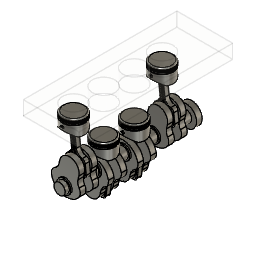
ic engine (Autodesk Fusion 360 design; units mm, degrees)
part number: 2025-07-07-10-14-35-876
part number: 2025-07-07-10-17-05-050
part number: 2025-07-07-10-17-21-308
part number: 2025-07-07-10-30-57-029
part number: 2025-07-07-10-31-19-349
part number: 2025-07-07-10-58-43-578
part number: 2025-07-07-10-58-53-469
part number: 2025-07-07-11-04-14-439
part number: 2025-07-07-15-54-50-928
part number: 2025-07-07-16-06-10-708
part number: 2025-07-07-16-45-22-649
Autodesk Fusion 360 part; units mm, degrees
note: some values were not read from the file. Set by a fixed rule: which face or edge a step refers to.
sketch "Sketch1" plane through (0, 0, 0) normal (0, 1, 0) x (1, 0, 0) in component "PISTON"
  line L0 (0, 0) -> (40, 0)
  line L1 (40, 0) -> (40, -55)
  line L2 (40, -55) -> (0, -55)
  line L3 (0, -55) -> (0, 0)
  line L4 (40, -48) -> (36, -48)
  line L5 (36, -48) -> (36, -46)
  line L6 (36, -46) -> (40, -46)
  line L7 (40, -46) -> (40, -48)
  line L8 (40, -44) -> (36, -44)
  line L9 (36, -44) -> (36, -42)
  line L10 (36, -42) -> (40, -42)
  line L11 (40, -42) -> (40, -44)
  line L12 (40, -38) -> (36, -38)
  line L13 (36, -38) -> (36, -36)
  line L14 (36, -36) -> (40, -36)
  line L15 (40, -36) -> (40, -38)
  dimension "d1" = 40
  dimension "d2" = 55
  dimension "d3" = 2
  dimension "d4" = 2
  dimension "d5" = 2
  dimension "d6" = 7
  dimension "d7" = 4
  dimension "d8" = 4
  dimension "d9" = 4
  dimension "d10" = 2
  dimension "d11" = 4
  constraint horizontal L0
  constraint vertical L1
  constraint horizontal L2
  constraint vertical L3
  constraint coincident L0.start L3.end
  constraint horizontal L4
  constraint vertical L5
  constraint horizontal L6
  constraint vertical L7
  constraint coincident L1 L4.start
  constraint horizontal L8
  constraint vertical L9
  constraint horizontal L10
  constraint vertical L11
  constraint coincident L1 L8.start
  constraint horizontal L12
  constraint vertical L13
  constraint horizontal L14
  constraint vertical L15
  constraint coincident L1 L12.start
  measures "d1" distance of L0.start L0.end
  measures "d2" distance of L0.start L2.end
  measures "d3" distance of L4.end L5.end
  measures "d4" distance of L8.end L9.end
  measures "d5" distance of L12.end L13.end
  measures "d6" distance of L2 L4
  measures "d7" distance of L4.start L4.end
  measures "d8" distance of L8.start L8.end
  measures "d9" distance of L12.start L12.end
  measures "d10" distance of L6 L8
  measures "d11" distance of L10 L12
revolve "Revolve1" add sketch "Sketch1" angle 360 about axis through (0, 0, 55) along (0, 0, -1) contours L0 L1 L2 L3 L4 L5 L6 L8 L9 L10 L12 L13 L14 makes body 1 in component "PISTON"
fillet "Fillet1" radius 5 1 edges at (-37.2931, -14.4646, 55) on bodies 1 in component "PISTON"
sketch "Sketch2" plane through (0, 0, 0) normal (0, 0, -1) x (1, 0, 0) in component "PISTON"
  circle A0 centre (0, 0) radius 40
  circle A1 centre (0, 0) radius 35
  dimension "d15" = 70
  constraint coincident A0.centre A1.centre
  measures "d15" diameter of A1
extrude "Extrude1" cut sketch "Sketch2" against normal blind 50 contours A1 bodies 1 in component "PISTON"
sketch "Sketch3" plane through (0, 0, 0) normal (0, 1, 0) x (1, 0, 0) in component "PISTON"
  line L0 (-40, 0) -> (40, 0)
  line L1 (-40, -36) -> (40, -36)
  line L2 (0, 0) -> (0, -13.6111)
  arc A0 (-35.5, 0) -> (35.5, 0) centre (0, 39.4894) ccw
  circle A1 centre (0, -24) radius 5
  dimension "d18" = 10
  dimension "d19" = 4.5
  dimension "d20" = 4.5
  dimension "d21" = 24
  constraint coincident L2.start origin
  constraint perpendicular L0 L2
  constraint coincident L2.end A0
  constraint coincident L0 A0.start
  constraint coincident L0 A0.end
  measures "d18" diameter of A1
  measures "d19" distance of L0.end A0.end
  measures "d20" distance of L0.start A0.start
  measures "d21" distance of L2.start A1.centre
extrude "Extrude2" cut sketch "Sketch3" along normal mid plane 80 bodies 1 in component "PISTON"
pattern_linear "00000000-0000-0000-0000-000000000000" [suppressed] in component "PISTONS"
sketch "Sketch1 (2)" plane through (0, 0, 0) normal (0, 1, 0) x (1, 0, 0) in component "connecting rod"
  circle A0 centre (0, -20) radius 5
  circle A1 centre (0, -20) radius 8.5
  circle A2 centre (0, 105) radius 22.5
  line L0 (-8.5, -20) -> (-8.5, 55)
  line L1 (0, 105) -> (-36, 105)
  line L2 (-36, 105) -> (-36, 80)
  line L3 (-36, 80) -> (-33.5, 80)
  line L4 (8.5, -20) -> (8.5, 55)
  line L5 (33.5, 80) -> (36, 80)
  line L6 (36, 80) -> (36, 105)
  line L7 (36, 105) -> (0, 105)
  arc A3 (-8.5, 55) -> (-33.5, 80) centre (-33.5, 55) ccw
  arc A4 (33.5, 80) -> (8.5, 55) centre (33.5, 55) ccw
  line L8 (36, 105) -> (-36, 105)
  line L9 (-36, 105) -> (-36, 137.5)
  line L10 (-36, 137.5) -> (36, 137.5)
  line L11 (36, 137.5) -> (36, 105)
  circle A5 centre (0, -5) radius 4.75
  circle A6 centre (0, 67.5) radius 4.75
  line L12 (4.75, -5) -> (4.75, 67.5)
  line L13 (-4.75, -5) -> (-4.75, 67.5)
  point P0 (8.5, 80)
  dimension "d28" = 10
  dimension "d29" = 17
  dimension "d30" = 45
  dimension "d31" = 125
  dimension "d32" = 36
  dimension "d33" = 25
  dimension "d34" = 27.5
  dimension "d35" = 25
  dimension "d36" = 72
  dimension "d37" = 32.5
  dimension "d38" = 9.5
  dimension "d39" = 9.5
  dimension "d40" = 15
  dimension "d41" = 37.5
  constraint concentric A0 A1
  constraint coincident A1 L0.start
  constraint tangent A1 L0
  constraint vertical L0
  constraint coincident A2.centre L1.start
  constraint horizontal L1
  constraint perpendicular L1 L2
  constraint perpendicular L2 L3
  constraint coincident A1 L4.start
  constraint tangent A1 L4
  constraint vertical L4
  constraint perpendicular L4 L5
  constraint perpendicular L5 L6
  constraint perpendicular L6 L7
  constraint tangent L3 A3
  constraint tangent L0 A3
  constraint coincident P0 L4
  constraint coincident P0 L5
  constraint tangent L4 A4
  constraint tangent L5 A4
  constraint equal A3 A4
  constraint horizontal L8
  constraint vertical L9
  constraint horizontal L10
  constraint vertical L11
  constraint coincident A5 L12.start
  constraint coincident A6 L12.end
  constraint tangent A6 L12
  constraint parallel L4 L12
  constraint coincident A5 L13.start
  constraint coincident A6 L13.end
  constraint tangent A6 L13
  constraint parallel L12 L13
  measures "d28" diameter of A0
  measures "d29" diameter of A1
  measures "d30" diameter of A2
  measures "d31" distance of A0.centre A2.centre
  measures "d32" distance of A2.centre L1.end
  measures "d33" distance of L1.end L2.end
  measures "d34" distance of P0 L5.end
  measures "d35" radius of A3
  measures "d36" distance of L6.end L1.end
  measures "d37" distance of L6.end L10.end
  measures "d38" diameter of A5
  measures "d39" diameter of A6
  measures "d40" distance of A0.centre A5.centre
  measures "d41" distance of A2.centre A6.centre
extrude "Extrude1'" add sketch "Sketch1 (2)" along normal mid plane 20 separate body contours A1 | A1 A2 L0 L1 L2 L3 L4 L5 L6 L7 A3 A4 L8 | A2 L1 L7 L8 L9 L10 L11 makes body 2 in component "connecting rod"
extrude "Extrude2'" add sketch "Sketch1 (2)" along normal mid plane 10 contours A5 | A5 A6 L12 L13 | A6 bodies 2 in component "connecting rod"
fillet "Fillet1'" radius 12.5 4 edges at (36, 0, -80) (36, 0, -137.5) (-36, 0, -137.5) (-36, 0, -80) on bodies 2 in component "connecting rod"
fillet "Fillet2" radius 2.5 24 edges at (0, 10, 28.5) (8.5, 10, -17.5) (13.6044, 10, -70.1383) (33.4478, 10, -83.573) (36, 10, -108.071) (32.3388, 10, -133.8388) (0, 10, -137.5) (-32.3388, 10, -133.8388) (-36, 10, -108.071) (-33.4478, 10, -83.573) (-13.6044, 10, -70.1383) (-8.5, 10, -17.5) (-33.4478, -10, -83.573) (-36, -10, -108.071) (-32.3388, -10, -133.8388) (0, -10, -137.5) (32.3388, -10, -133.8388) (36, -10, -108.071) (33.4478, -10, -83.573) (13.6044, -10, -70.1383) (8.5, -10, -17.5) (0, -10, 28.5) (-8.5, -10, -17.5) (-13.6044, -10, -70.1383) on bodies 2 in component "connecting rod"
cylinder "CylinderPrimitive1" add diameter 10 height -90 placed x (1, 0, 0) y (0, 0, -1) z (0, 1, 0) at (50, 0, 25) separate body makes body 3 in component "pin"
fillet "Fillet1''" radius 1.5 2 edges at (51.8081, 0, 29.6616) (48.1919, -90, 29.6616) on bodies 3 in component "pin"
pattern_linear "00000000-0000-0000-0000-000000000000'" [suppressed] in component "pins"
sketch "Sketch1 (3)" plane through (0, 0, 0) normal (0, 1, 0) x (1, 0, 0) in component "crankshafts"
  circle A0 centre (0, 105) radius 22.5
  circle A1 centre (0, 105) radius 35
  circle A2 centre (0, 40.5) radius 20
  circle A3 centre (0, 40.5) radius 25
  arc A4 (-55, 62.5) -> (55, 62.5) centre (0, 62.5) ccw
  line L0 (-35, 105) -> (-35, 62.5)
  line L1 (35, 105) -> (35, 62.5)
  line L2 (-35, 62.5) -> (-55, 62.5)
  line L3 (35, 62.5) -> (55, 62.5)
  dimension "d63" = 70
  dimension "d64" = 110
  dimension "d65" = 40
  dimension "d66" = 50
  dimension "d67" = 42.5
  dimension "d68" = 22
  constraint concentric A0 A1
  constraint concentric A2 A3
  constraint coincident A1 L0.start
  constraint tangent A1 L0
  constraint coincident A1 L1.start
  constraint tangent A1 L1
  measures "d63" diameter of A1
  measures "d64" diameter of A4
  measures "d65" diameter of A2
  measures "d66" diameter of A3
  measures "d67" distance of A0.centre A4.centre
  measures "d68" distance of A4.centre A2.centre
extrude "Extrude1''" add sketch "Sketch1 (3)" along normal blind 20 from surface at 15 separate body contours A0 | A1 | A1 A4 L0 L1 L2 L3 | A2 | A3 makes body 4 in component "crankshafts"
extrude "Extrude2''" add sketch "Sketch1 (3)" against normal blind 20 from surface at 15 contours A2 bodies 4 in component "crankshafts"
extrude "Extrude3" add sketch "Sketch1 (3)" against normal blind 5 from surface at 15 contours A3 bodies 4 in component "crankshafts"
fillet "Fillet1'''" radius 30 2 edges at (35, 25, -62.5) (-35, 25, -62.5) on bodies 4 in component "crankshafts"
fillet "Fillet2'" radius 25 2 edges at (-55, 25, -62.5) (55, 25, -62.5) on bodies 4 in component "crankshafts"
mirror "Mirror1" about plane through (0, 48, 0) normal (0, 1, 0) of bodies 4 makes body 5 in component "crankshafts"
extrude "Extrude4" add sketch "Sketch1 (3)" along normal blind 61 contours A0 bodies 4 5 in component "crankshafts"
extrude "Extrude5" cut sketch "Sketch1 (3)" along normal blind 15 contours A0 bodies 4 in component "crankshafts"
pattern_linear "R-Pattern1" count 4 spacing 105.6667 along (0, -1, 0) of bodies 4 makes body 6 at (-29.6043, -70.6667, -60.6489) makes body 7 at (-29.6043, -176.3333, -60.6489) makes body 8 at (-29.6043, -282, -60.6489) in component "crankshafts"
move_body "Move1" bodies 7 6 to x (-1, 0, 0) y (0, 1, 0) z (0, 0, -1) at (0, 0, -81) in component "crankshafts"
combine "Combine1" operation add target body 7 tool bodies 8 4 6 in component "crankshafts"
extrude "Extrude6" add 1 faces at (1.2228, 101, -45.27) along direction (0, 1, 0) blind 50 on bodies 7 bodies 7 in component "crankshafts"
sketch "Sketch1 (4)" plane through (0, 103, 0) normal (0, 1, 0) x (-1, 0, 0)
  circle A0 centre (0, -40.5) radius 20
  circle A1 centre (0, -40.5) radius 37.5
  dimension "d94" = 75
  constraint concentric A0 A1
  measures "d94" diameter of A1
extrude "Extrude1'''" add sketch "Sketch1 (4)" against normal blind 20 separate body makes body 9 in component "Component"
sketch "Sketch2 (2)" plane through (-1.0737, 0, 179.9687) normal (-0.005966, 0, 0.999982) x (0, -1, 0)
sketch "Sketch3 (2)" plane through (0, 0, 51) normal (0, 0, 1) x (-1, 0, 0)
  circle A0 centre (0, 2.9976) radius 35
  line L0 (100, -150) -> (-100, -150)
  line L1 (-100, -150) -> (-100, 400)
  line L2 (-100, 400) -> (100, 400)
  line L3 (100, 400) -> (100, -150)
  circle A1 centre (0, 2.9976) radius 40
  circle A2 centre (0, 102.6643) radius 40
  circle A3 centre (-2.1816, 214.3309) radius 40
  circle A4 centre (0, 319.9976) radius 40
  constraint horizontal L0
  constraint vertical L1
  constraint horizontal L2
  constraint vertical L3
extrude "Extrude1''''" add sketch "Sketch3 (2)" along normal blind 25 separate body contours L0 L1 L2 L3 makes body 10 in component "Component''"
extrude "Extrude2'''" add 1 faces at (-0.9964, 112.2969, 76) along direction (0, 0, 1) blind 125 on bodies 10 bodies 10 in component "Component''"
extrude "Extrude1'''''" cut 1 faces at (-0.9964, 112.2969, 51) faces seen with x (1, 0, 0) y (0, 1, 0) z (0, 0, 1) at (50, 57.6667, -124) along direction (0, 0, 1) blind 100 on bodies 10 bodies 3 in component "pin"
extrude "Extrude7" cut 1 faces at (-0.9964, 112.2969, 51) faces seen with x (1, 0, 0) y (0, 1, 0) z (0, 0, 1) at (0, 48, 0) along direction (0, 0, 1) blind 100 on bodies 10 bodies 7 in component "crankshafts"
extrude "Extrude3'" cut 1 faces at (-0.9964, 112.2969, 51) along direction (0, 0, 1) blind 100 on bodies 10 bodies 10 in component "Component''"
component "connecting rods" placed x (-1, 0, 0) y (0, -1, 0) z (0, 0, 1) at (0, -3, 129)
component "pins" placed x (1, 0, 0) y (0, 1, 0) z (0, 0, 1) at (0, 0, 0)
component "crankshafts" placed x (-1, 0, 0) y (0, 1, 0) z (0, 0, -1) at (0, -48, -81)
component "PISTONS" placed x (1, 0, 0) y (0, 1, 0) z (0, 0, 1) at (0, 0, 0)
component "Component" placed x (1, 0, 0) y (0, 1, 0) z (0, 0, 1) at (0, 0, 0)
component "connecting rod" placed x (-1, 0, 0) y (0, -1, 0) z (0, 0, 1) at (0, -102.6667, 0)
component "connecting rod" placed x (-0.999848, 0, 0.017452) y (0, -1, 0) z (0.017452, 0, 0.999848) at (1.8325, -214.3333, -0.016)
component "connecting rod" placed x (1, 0, 0) y (0, 1, 0) z (0, 0, 1) at (0, -320, 129)
component "Component''" placed x (1, 0, 0) y (0, 1, 0) z (0, 0, 1) at (0, 0, 0)
component "PISTON" placed x (1, 0, 0) y (0, 1, 0) z (0, 0, 1) at (0, -2.9976, 125) in component "PISTONS"
component "PISTON" placed x (1, 0, 0) y (0, 1, 0) z (0, 0, 1) at (0, -102.6643, -4) in component "PISTONS"
component "PISTON" placed x (1, 0, 0) y (0, 1, 0) z (0, 0, 1) at (2.1816, -214.3309, -4.019) in component "PISTONS"
component "PISTON" placed x (1, 0, 0) y (0, 1, 0) z (0, 0, 1) at (0, -319.9976, 125) in component "PISTONS"
component "connecting rod" placed x (1, 0, 0) y (0, 1, 0) z (0, 0, 1) at (0, 0, 0) in component "connecting rods"
component "Component'" placed x (1, 0, 0) y (0, 1, 0) z (0, 0, 1) at (0, 0, 0) in component "connecting rod"
component "pin" placed x (1, 0, 0) y (0, 1, 0) z (0, 0, 1) at (-50, 42, 124) in component "pins"
component "pin" placed x (1, 0, 0) y (0, 1, 0) z (0, 0, 1) at (-50, -57.6667, -5) in component "pins"
component "pin" placed x (1, 0, 0) y (0, 1, 0) z (0, 0, 1) at (-50, -275, 124) in component "pins"
component "pin" placed x (-0.93358, 0, -0.358368) y (0, 1, 0) z (0.358368, 0, -0.93358) at (39.9014, -169.3333, 61.2389) in component "pins"
